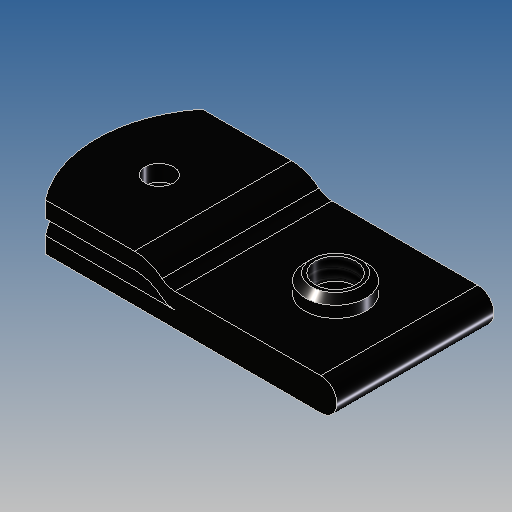
# Autodesk Inventor part: End Resistor Peice
Saved by Autodesk Inventor 2018 (Build 220112000, 112)
## iProperties
Created: 2018-02-23
Part Number: End Resistor Peice
Material: Stainless Steel
Document SubType Name: Modeling
Designer: 232963
Density: 8 g/cm^3
Appearance: Semi-Polished
Mass: 45.5302 g
Surface Area: 44.2126 cm^2
Volume: 5.69128 cm^3
Author: 232963
Autodesk Inventor part; units mm, degrees
ref_plane "YZ Plane" through (0, 0, 0) normal (1, 0, 0) x (0, 1, 0)
ref_plane "XZ Plane" through (0, 0, 0) normal (0, 1, 0) x (-1, 0, 0)
ref_plane "XY Plane" through (0, 0, 0) normal (0, 0, 1) x (1, 0, 0)
sketch "Sketch1" plane through (0, 0, 0) normal (0, 0, 1) x (1, 0, 0)
  line L0 (-16.1963, 11.291) -> (2.06, 11.291)
  line L1 (33.81, 9.005) -> (33.81, 3.925)
  line L2 (33.81, 3.925) -> (-16.1963, 3.925)
  line L3 (33.81, 9.005) -> (8.411, 9.005)
  line L4 (-16.1963, 11.291) -> (2.06, 11.291)
  arc A0 (6.3875, 9.7333) -> (2.06, 11.291) centre (2.06, 4.5007) ccw
  line L5 (-16.1963, 8.751) -> (2.06, 8.751)
  arc A1 (6.3875, 7.1933) -> (2.06, 8.751) centre (2.06, 1.9607) ccw
  arc A2 (6.3875, 9.7333) -> (8.411, 9.005) centre (8.411, 12.18) ccw
  line L6 (8.411, 6.465) -> (8.5599, 6.465)
  arc A3 (6.3875, 7.1933) -> (8.411, 6.465) centre (8.411, 9.64) ccw
  line L7 (-16.1963, 6.465) -> (8.411, 6.465)
  line L8 (-16.1963, 3.925) -> (-16.1963, 6.465)
  line L9 (-16.1963, 8.751) -> (-16.1963, 11.291)
  point P0 (0, 0)
  point P1 (7.1412, 9.005)
  point P2 (7.1412, 6.465)
  dimension "d2" = 5.08
  dimension "d7" = 2.54
  dimension "d8" = 0
  dimension "d9" = 2.54
  dimension "d10" = 0
  dimension "d11" = 3.175
  dimension "d12" = 3.175
  dimension "d58" = 7.366
  constraints: 20 end point, 11 point on circle, 5 tangent, 4 centre point, 3 horizontal, 3 parallel, 2 perpendicular, 2 point on line
  measures "d2" distance between parallel lines of L2 L3
  measures "d7" distance from line of point (7.141, 6.465) L3
  measures "d8" horizontal distance of point (7.141, 9.005) point (7.141, 6.465)
  measures "d9" distance between centres of A0 A1
  measures "d10" horizontal distance of L5.end L0.end
  measures "d11" radius of A2
  measures "d12" radius of A3
  measures "d58" distance between parallel lines of L0 L2
extrude "Extrusion1" add sketch "Sketch1" along normal blind 24.6062
sketch "Sketch2" plane through (0, 0, 24.6062) normal (0, 0, 1) x (1, 0, 0)
  line L0 (-16.1963, 3.925) -> (33.81, 3.925) projected
  line L1 (33.81, 9.005) -> (8.411, 9.005) projected
  arc A0 (31.27, 3.925) -> (31.27, 9.005) centre (31.27, 6.465) ccw
  line L2 (33.81, 3.925) -> (33.81, 9.005) projected
  point P0 (0, 0)
  dimension "d17" = 0
  constraints: 2 point on circle, 2 point on line, 2 tangent, 1 centre point
  measures "d17" distance edge to line of A0 L2
extrude "Extrusion2" cut sketch "Sketch2" against normal blind 24.6062 fills toward (33.86, 6.465) open curves A0
sketch "Sketch3" plane through (-16.1963, 11.291, 0) normal (0, 1, 0) x (1, 0, 0)
  line L0 (18.2563, 0) -> (0, 0) projected
  line L1 (0, -24.6062) -> (47.4663, -24.6062) projected
  arc A0 (4.2862, 0) -> (4.2862, -24.6062) centre (19.8004, -12.3031) ccw
  line L2 (0, 0) -> (0, -24.6062) projected
  line L3 (18.2563, 0) -> (18.2563, -24.6062) projected
  point P0 (16.1963, 0)
  dimension "d21" = 13.97
  dimension "d22" = 13.97
  constraints: 2 point on circle, 2 point on line, 1 centre point, 1 tangent
  measures "d21" distance from line of A0.end L3
  measures "d22" distance from line of L3 A0.start
extrude "Extrusion3" cut sketch "Sketch3" against normal blind 8.7313 contours A0 L2 L0 | A0 L1 L2
sketch "Sketch4" plane through (8.411, 9.005, 24.6062) normal (0, 1, 0) x (1, 0, 0)
  line L0 (25.399, 24.6062) -> (25.399, 0) projected
  line L1 (22.859, 0) -> (0, 0) projected
  point P0 (-8.411, 24.6062)
  point P1 (12.8641, 12.3031)
  dimension "d25" = 12.5349
  dimension "d26" = 24.6062
  dimension "d27" = 12.3031
  measures "d25" distance from line of point (12.864, 12.303) L0
  measures "d26" distance of L0.start L0.end
  measures "d27" distance from line of L1 point (12.864, 12.303)
hole "Hole1" at (21.2751, 9.005, 12.3031) direction (0, -1, 0) diameter 6.4008 end through all thread size "5/16-18 UNC" class "2B" standard "ANSI Unified Screw Threads"
sketch "Sketch5" plane through (31.27, 3.925, 0) normal (0, -1, 0) x (1, 0, 0)
  circle A0 centre (-9.9949, 12.3031) radius 3.2004 projected
  point P0 (-31.27, 0)
  constraints: 1 coincident
hole "Hole2" at (21.2751, 3.925, 12.3031) direction (0, 1, 0) diameter 9.906 depth 3.429 tip angle 118
sketch "Sketch6" plane through (8.411, 9.005, 24.6062) normal (0, 1, 0) x (1, 0, 0)
  circle A0 centre (12.8641, 12.3031) radius 3.2004 projected
  circle A1 centre (12.8641, 12.3031) radius 4.7879
  point P0 (-8.411, 24.6062)
  dimension "d42" = 1.5875
  constraints: 1 centre point, 1 coincident
  measures "d42" radial gap between concentric circles of A0 A1
extrude "Extrusion4" add sketch "Sketch6" along normal blind 2.794
chamfer "Chamfer1" distance 1.016 angle 45 1 edges at (16.4872, 11.799, 12.3031)
sketch "Sketch7" plane through (2.06, 11.291, 24.6062) normal (0, 1, 0) x (1, 0, 0)
  line L0 (-2.06, 24.6062) -> (-2.06, 0)
  line L1 (6.351, 0) -> (-13.97, 0) projected
  point P0 (-8.41, 12.3031)
  dimension "d48" = 6.35
  dimension "d49" = 24.6062
  dimension "d50" = 12.3031
  constraints: 2 end point, 1 point on line, 1 vertical
  measures "d48" distance from line of L0 point (-8.41, 12.303)
  measures "d49" distance of L0.start L0.end
  measures "d50" distance from line of L1 point (-8.41, 12.303)
hole "Hole3" at (-6.35, 11.291, 12.3031) direction (0, -1, 0) diameter 4.445 end through all
equation "\"d27\" = 0.5 * d26"
equation "\"d50\" = 0.5 * d49"
body "Solid1"
